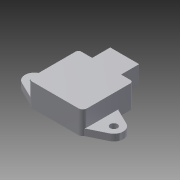
# Autodesk Inventor part: Bosch TPS
Saved by Autodesk Inventor 2015 (Build 190159000, 159)
## iProperties
Created: 2015-08-27
Part Number: Bosch TPS
Material: PC/ABS Plastic
Description: insert part description/title
Document SubType Name: Modeling
Designer: c3148102
Density: 0.357273 g/cm^3
Appearance: Smooth - White
Part Category: insert part category here and press enter to fill value
Author: c3148102
Autodesk Inventor part; units mm, degrees
ref_plane "YZ Plane" through (0, 0, 0) normal (1, 0, 0) x (0, 1, 0)
ref_plane "XZ Plane" through (0, 0, 0) normal (0, 1, 0) x (-1, 0, 0)
ref_plane "XY Plane" through (0, 0, 0) normal (0, 0, 1) x (1, 0, 0)
sketch "Sketch1" plane through (0, 0, 0) normal (0, 0, 1) x (1, 0, 0)
  line L0 (-56.4878, 0) -> (56.4878, 0) construction
  line L1 (0, 20.952) -> (0, -20.952) construction
  line L2 (-19, 15.5) -> (-19, -14.5)
  line L3 (19, 15.5) -> (19, -14.5)
  line L4 (-17, 17.5) -> (17, 17.5)
  line L5 (-16, -17.5) -> (16, -17.5)
  arc A0 (19, 15.5) -> (17, 17.5) centre (17, 15.5) ccw
  arc A1 (-17, 17.5) -> (-19, 15.5) centre (-17, 15.5) ccw
  arc A2 (16, -17.5) -> (19, -14.5) centre (16, -14.5) ccw
  arc A3 (-19, -14.5) -> (-16, -17.5) centre (-16, -14.5) ccw
  circle A4 centre (-27.5, -4.5) radius 2.25
  circle A5 centre (27.5, -4.5) radius 2.5
  arc A6 (-30.3494, 1.3422) -> (-30.3494, -10.3422) centre (-27.5, -4.5) ccw
  line L6 (-30.3494, -10.3422) -> (-18.5349, -16.1045)
  line L7 (-30.3494, 1.3422) -> (-19.5616, 6.6037)
  arc A7 (-19.5616, 6.6037) -> (-19, 7.5025) centre (-20, 7.5025) ccw
  line L8 (-27.5, -4.5) -> (27.5, -4.5) construction
  arc A8 (30.3494, -10.3422) -> (30.3494, 1.3422) centre (27.5, -4.5) ccw
  line L9 (19.5616, 6.6037) -> (30.3494, 1.3422)
  line L10 (18.5349, -16.1045) -> (30.3494, -10.3422)
  arc A9 (19, 7.5025) -> (19.5616, 6.6037) centre (20, 7.5025) ccw
  point P0 (0, 0)
  point P1 (0, 0)
  point P2 (-19, -17.5)
  point P3 (-19, 0)
  point P4 (19, -17.5)
  point P5 (-19, 17.5)
  point P6 (19, 17.5)
  dimension "d0" = 38
  dimension "d1" = 35
  dimension "d2" = 55
  dimension "d3" = 2
  dimension "d4" = 3
  dimension "d5" = 13
  dimension "d6" = 4.5
  dimension "d7" = 5
  dimension "d8" = 13
  dimension "d12" = 2
  dimension "d13" = 26
  dimension "d14" = 26
  dimension "d15" = 13
  dimension "d16" = 26
  dimension "d17" = 26
  dimension "d18" = 2
  constraints: 22 end point, 18 point on circle, 16 tangent, 10 centre point, 10 point on line, 5 coincident, 2 equal radius, 2 horizontal, 2 midpoint, 2 parallel, 1 symmetric about line, 1 vertical, 2 other
  measures "d0" distance between parallel lines of L3 L2
  measures "d1" distance between parallel lines of L5 L4
  measures "d2" distance of point (27.5, -4.5) point (-27.5, -4.5)
  measures "d3" radius of A0
  measures "d4" radius of A2
  measures "d5" distance from line of point (-27.5, -4.5) L5
  measures "d6" diameter of A4
  measures "d7" diameter of A5
  measures "d8" diameter of A6
  measures "d12" diameter of A7
  measures "d13" angle of L8 L7
  measures "d14" angle of L6 L8
  measures "d15" diameter of A8
  measures "d16" angle of L8 L9
  measures "d17" angle of L10 L8
  measures "d18" diameter of A9
extrude "Extrusion1" add sketch "Sketch1" along normal blind 4.6
extrude "Extrusion2" add sketch "Sketch1" along normal blind 16 contours A1 L4 A0 L3 A2 L5 A3 L2
sketch "Sketch2" plane through (0, 0, 0) normal (0, 0, -1) x (-1, 0, 0)
  line L0 (0, 53.517) -> (0, -53.517) construction
  circle A0 centre (-27.5, -4.5) radius 2.5 construction
  circle A1 centre (27.5, -4.5) radius 2.25 construction
  line L1 (-27.5, -4.5) -> (27.5, -4.5) construction
  line L2 (-3, 31.057) -> (-3, -31.9192) construction
  line L3 (-19, 7.5025) -> (-19, 15.5) construction
  circle A2 centre (-3, -4.5) radius 7.55
  point P0 (0, 0)
  point P1 (0, 0)
  dimension "d24" = 16
  dimension "d25" = 15.1
  constraints: 6 end point, 2 point on line, 1 centre point, 1 coincident, 1 horizontal, 1 midpoint, 1 parallel, 1 vertical
  measures "d24" distance between parallel lines of L3 L2
  measures "d25" diameter of A2
extrude "Extrusion3" add sketch "Sketch2" along normal blind 2
chamfer "Chamfer1" distance 0.5 angle 45 1 edges at (10.55, -4.5, -2)
sketch "Sketch3" plane through (3, -4.5, -2) normal (0, 0, -1) x (-1, 0, 0)
  circle A0 centre (0, 0) radius 7.05 projected
  line L0 (-15.8826, 0) -> (15.8826, 0) construction
  line L1 (0, 11.2082) -> (0, -11.2082) construction
  arc A1 (-3.4641, 2) -> (3.4641, 2) centre (0, 0) ccw
  line L2 (3.4641, 2) -> (-3.4641, 2)
  circle A2 centre (0, 0) radius 4
  point P0 (3, 4.5)
  dimension "d31" = 8
  dimension "d33" = 2
  dimension "d43" = 8
  constraints: 6 end point, 3 coincident, 2 centre point, 2 midpoint, 2 point on circle, 1 horizontal, 1 parallel, 1 vertical
  measures "d31" diameter of A1
  measures "d33" distance between parallel lines of L0 L2
  measures "d43" diameter of A2
extrude "Extrusion4" cut sketch "Sketch3" against normal blind 12 contours L2 A1
sketch "Sketch4" plane through (-17, 17.5, 0) normal (0, 1, 0) x (1, 0, 0)
  line L0 (34, -16) -> (0, -16) projected
  line L1 (34, 0) -> (0, 0) projected
  line L2 (34, 0) -> (34, -16) projected
  line L3 (0, 0) -> (0, -16) projected
  line L4 (17, -16) -> (17, 0) construction
  line L5 (34, -9.7) -> (0, -9.7) construction
  line L6 (27, -16) -> (27, -3.4)
  line L7 (7, -16) -> (7, -3.4)
  line L8 (27, -16) -> (7, -16)
  line L9 (27, -3.4) -> (7, -3.4)
  point P0 (27, -9.7)
  dimension "d39" = 9.7
  dimension "d40" = 20
  constraints: 12 end point, 4 point on line, 3 parallel, 2 midpoint, 2 symmetric about line, 1 collinear, 1 perpendicular
  measures "d39" distance between parallel lines of L1 L5
  measures "d40" distance between parallel lines of L7 L6
extrude "Extrusion5" add sketch "Sketch4" along normal blind 13 contours L0 L7 L9 L6
extrude "Extrusion6" cut sketch "Sketch3" against normal blind 6 contours A2 L2
chamfer "Chamfer3" distance 1 distance2 1.99 1 edges at (3, -2.5, 4) measured on face at (3, -2.5, 4.5)
sketch "Sketch5" plane through (0, 0, 16) normal (0, 0, 1) x (1, 0, 0)
  line L0 (10, 17.5) -> (10, 30.5) projected
  line L1 (-10, 30.5) -> (10, 30.5) projected
  line L2 (-10, 17.5) -> (-10, 30.5) projected
  line L3 (10, 30.5) -> (-10, 30.5)
  line L4 (-10, 30.5) -> (-10, 17.5)
  line L5 (-10, 17.5) -> (10, 17.5)
  line L6 (10, 17.5) -> (10, 30.5)
  point P0 (0, 0)
  constraints: 8 end point, 2 parallel, 1 horizontal, 1 perpendicular
extrude "Extrusion7" cut sketch "Sketch5" against normal blind 0.5
equation "\"d14\" = d13"
equation "\"d16\" = d13"
equation "\"d17\" = d13"
body "Solid1"
